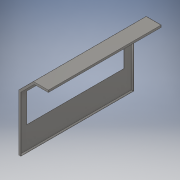
# Autodesk Inventor part: Front Panel
Saved by Autodesk Inventor 2018 (Build 220112000, 112)
## iProperties
Created: 2018-08-09
Part Number: Front Panel
Material: Steel
Document SubType Name: Modeling
Designer: P301319
Density: 7.85 g/cm^3
Appearance: Stainless - Brushed
Author: P301319
Autodesk Inventor part; units mm, degrees
ref_plane "YZ Plane" through (0, 0, 0) normal (1, 0, 0) x (0, 1, 0)
ref_plane "XZ Plane" through (0, 0, 0) normal (0, 1, 0) x (-1, 0, 0)
ref_plane "XY Plane" through (0, 0, 0) normal (0, 0, 1) x (1, 0, 0)
sketch "Sketch1" plane through (0, 0, 0) normal (0, 0, 1) x (1, 0, 0)
  line L0 (150, 800) -> (304, 800)
  line L1 (150, 800) -> (0, 650)
  line L2 (150, 800) -> (1016.5277, 800) construction
  line L3 (0, 650) -> (0, 70)
  line L4 (1.6, 70) -> (1.6, 649.3373)
  line L5 (1.6, 649.3373) -> (150.6627, 798.4)
  line L6 (150.6627, 798.4) -> (304, 798.4)
  line L7 (304, 800) -> (304, 798.4)
  line L8 (0, 70) -> (1.6, 70)
  point P0 (0, 0)
  dimension "d0" = 154
  dimension "d1" = 800
  dimension "d2" = 135
  dimension "d8" = 150
  dimension "d9" = 580
  dimension "d10" = 70
  dimension "d19" = 1.6
  constraints: 18 end point, 3 horizontal, 1 perpendicular, 1 vertical, 2 other
  measures "d0" distance of L0.start L0.end
  measures "d1" distance from line of point (0, 0) L0
  measures "d2" angle of L1 L2
  measures "d8" horizontal distance of point (0, 0) L0.start
  measures "d9" distance of L1.end L3.end
  measures "d10" distance of point (0, 0) L3.end
  measures "d19" distance between parallel lines of L1 L5
extrude "Extrusion1" add sketch "Sketch1" along normal blind 1160
sketch "Sketch2" plane through (0, 70, 0) normal (-1, 0, 0) x (0, 0, 1)
  line L0 (80, 530) -> (1080, 530)
  line L1 (1080, 530) -> (1080, 230)
  line L2 (1080, 230) -> (80, 230)
  line L3 (80, 230) -> (80, 530)
  line L4 (0, 0) -> (0, 580) projected
  line L5 (0, 580) -> (1160, 580) projected
  line L6 (0, 0) -> (1160, 0) projected
  point P0 (0, -70)
  point P1 (580, 230)
  point P2 (580, 0)
  dimension "d13" = 1000
  dimension "d14" = 300
  dimension "d16" = 50
  constraints: 8 end point, 2 midpoint, 2 parallel, 1 horizontal, 1 perpendicular, 1 vertical alignment
  measures "d13" distance of L1.end L2.end
  measures "d14" distance of L0.end L1.end
  measures "d16" distance between parallel lines of L5 L0
extrude "Extrusion2" cut sketch "Sketch2" against normal through all
sketch "Sketch3" plane through (0, 0, 1160) normal (0, 0, 1) x (1, 0, 0)
  line L0 (150.6627, 798.4) -> (304, 798.4) projected
  line L1 (1.6, 649.3373) -> (150.6627, 798.4) projected
  line L2 (1.6, 70) -> (1.6, 649.3373) projected
  line L3 (304, 778.4) -> (158.947, 778.4)
  line L4 (158.947, 778.4) -> (21.6, 641.053)
  line L5 (21.6, 641.053) -> (21.6, 70)
  line L6 (304, 778.4) -> (304, 798.4)
  line L7 (304, 800) -> (150, 800) projected
  line L8 (21.6, 70) -> (1.6, 70)
  point P0 (0, 0)
  dimension "d20" = 20
  constraints: 10 end point, 1 horizontal, 1 perpendicular, 2 other
  measures "d20" distance between parallel lines of L1 L4
extrude "Extrusion3" add sketch "Sketch3" against normal blind 1.6
sketch "Sketch4" plane through (0, 0, 0) normal (0, 0, -1) x (-1, 0, 0)
  line L0 (-304, 798.4) -> (-150.6627, 798.4) projected
  line L1 (-304, 798.4) -> (-304, 778.4) projected
  line L2 (-304, 778.4) -> (-158.947, 778.4) projected
  line L3 (-158.947, 778.4) -> (-21.6, 641.053) projected
  line L4 (-21.6, 641.053) -> (-21.6, 70) projected
  line L5 (-21.6, 70) -> (-1.6, 70) projected
  line L6 (-1.6, 649.3373) -> (-1.6, 70) projected
  line L7 (-150.6627, 798.4) -> (-1.6, 649.3373) projected
  point P0 (0, 0)
extrude "Extrusion4" add sketch "Sketch4" against normal blind 1.6
sketch "Sketch5" plane through (304, 800, 1160) normal (1, 0, 0) x (0, 0, -1)
  line L0 (1158.4, -1.6) -> (1.6, -1.6) projected
  line L1 (1158.4, -21.6) -> (1158.4, -1.6) projected
  line L2 (1.6, -1.6) -> (1.6, -21.6) projected
  line L3 (1.6, -21.6) -> (1.6, -158.947) projected
  line L4 (1.6, -21.6) -> (1158.4, -21.6)
  point P0 (1160, -800)
  constraints: 2 end point, 1 perpendicular
extrude "Extrusion5" add sketch "Sketch5" against normal blind 1.6
sketch "Sketch6" plane through (0, 70, 0) normal (0, -1, 0) x (1, 0, 0)
  line L0 (1.6, 1.6) -> (21.6, 1.6) projected
  line L1 (1.6, 1.6) -> (1.6, 1158.4) projected
  line L2 (21.6, 1158.4) -> (1.6, 1158.4) projected
  line L3 (158.947, 1158.4) -> (21.6, 1158.4) projected
  line L4 (21.6, 1.6) -> (21.6, 1158.4)
  point P0 (0, 0)
  constraints: 2 end point, 1 vertical
extrude "Extrusion6" add sketch "Sketch6" against normal blind 1.6
sketch "Sketch7" plane through (304, 800, 1160) normal (1, 0, 0) x (0, 0, -1)
  line L0 (1.6, -1.6) -> (1.6, -21.6) projected
  line L1 (1.6, -1.6) -> (3.2, -1.6)
  line L2 (3.2, -1.6) -> (3.2, -21.6)
  line L3 (3.2, -21.6) -> (1.6, -21.6)
  line L4 (1.6, -21.6) -> (1.6, -1.6)
  line L5 (1158.4, -21.6) -> (1158.4, -1.6) projected
  line L6 (1158.4, -1.6) -> (1156.8, -1.6)
  line L7 (1156.8, -1.6) -> (1156.8, -21.6)
  line L8 (1156.8, -21.6) -> (1158.4, -21.6)
  line L9 (1158.4, -21.6) -> (1158.4, -1.6)
  point P0 (1160, -800)
  dimension "d32" = 1.6
  dimension "d33" = 20
  dimension "d34" = 1.6
  dimension "d35" = 20
  constraints: 16 end point, 4 parallel, 2 horizontal, 2 perpendicular
  measures "d32" distance of L2.end L3.end
  measures "d33" distance of L1.end L2.end
  measures "d34" distance of L8.end L7.end
  measures "d35" distance of L7.end L6.end
extrude "Extrusion7" cut sketch "Sketch7" against normal blind 1.6
sketch "Sketch8" plane through (0, 70, 0) normal (0, -1, 0) x (1, 0, 0)
  line L0 (1.6, 1158.4) -> (1.6, 1.6) projected
  line L1 (1.6, 1.6) -> (21.6, 1.6)
  line L2 (21.6, 1.6) -> (21.6, 3.2)
  line L3 (21.6, 3.2) -> (1.6, 3.2)
  line L4 (1.6, 3.2) -> (1.6, 1.6)
  line L5 (1.6, 1158.4) -> (21.6, 1158.4)
  line L6 (21.6, 1158.4) -> (21.6, 1156.8)
  line L7 (21.6, 1156.8) -> (1.6, 1156.8)
  line L8 (1.6, 1156.8) -> (1.6, 1158.4)
  point P0 (0, 0)
  dimension "d38" = 20
  dimension "d39" = 1.6
  dimension "d40" = 20
  dimension "d41" = 1.6
  constraints: 16 end point, 4 parallel, 2 horizontal, 2 perpendicular
  measures "d38" distance of L3.end L2.end
  measures "d39" distance of L2.end L1.end
  measures "d40" distance of L6.end L7.end
  measures "d41" distance of L5.end L6.end
extrude "Extrusion8" cut sketch "Sketch8" against normal blind 1.6
body "Solid1"
